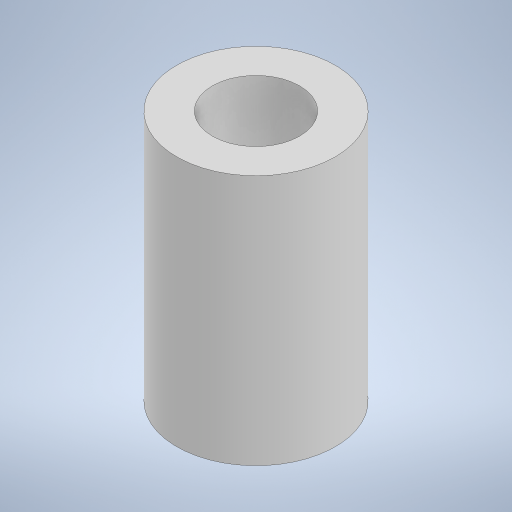
# Autodesk Inventor part: Деталь1
Saved by Autodesk Inventor 2024 (Build 280153000, 153)
## iProperties
Created: 2024-04-27
Part Number: Деталь1
Material: Типовые
Document SubType Name: Modeling
Designer: stefa
Density: 1 g/cm^3
Appearance: По умолчанию
Author: stefa
Autodesk Inventor part; units mm, degrees
ref_plane "YZ Plane" through (0, 0, 0) normal (1, 0, 0) x (0, 1, 0)
ref_plane "XZ Plane" through (0, 0, 0) normal (0, 1, 0) x (-1, 0, 0)
ref_plane "XY Plane" through (0, 0, 0) normal (0, 0, 1) x (1, 0, 0)
sketch "Эскиз1" plane through (0, 0, 0) normal (0, 1, 0) x (-1, 0, 0)
  circle A0 centre (0, 0) radius 12.7
  circle A1 centre (0, 0) radius 15
  dimension "d0" = 25.4
  dimension "d1" = 30
  constraints: 2 centre point, 2 coincident
  measures "d0" diameter of A0
  measures "d1" diameter of A1
extrude "Выдавливание1" add sketch "Эскиз1" along normal blind 17.5
sketch "Эскиз3" plane through (0, 17.5, 0) normal (0, 1, 0) x (1, 0, 0)
  circle A0 centre (0, 0) radius 15
  circle A1 centre (0, 0) radius 8.25
  circle A2 centre (0, 0) radius 15 projected
  dimension "d4" = 16.5
  dimension "d9" = 0
  constraints: 2 centre point, 2 coincident
  measures "d4" diameter of A1
  measures "d9" radial gap between concentric circles of A2 A0
extrude "Выдавливание2" add sketch "Эскиз3" along normal blind 30
fillet "Сопряжение1" radius 5 1 edges at (-8.25, 17.5, 0)
fillet "Сопряжение2" radius 1 2 edges at (0, 17.5, -12.7) (0, 17.5, 12.7)
